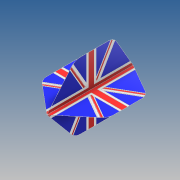
# Autodesk Inventor part: Millan Dart Flight
Saved by Autodesk Inventor 2018.2 (Build 222227000, 227)
## iProperties
Created: 2018-01-12
Part Number: Millan Dart Flight
Material: Generic
Document SubType Name: Modeling
Designer: Thomas Savage
Density: 1 g/cm^3
Appearance: Default
Author: Thomas Savage
Autodesk Inventor part; units mm, degrees
ref_plane "YZ Plane" through (0, 0, 0) normal (1, 0, 0) x (0, 1, 0)
ref_plane "XZ Plane" through (0, 0, 0) normal (0, 1, 0) x (-1, 0, 0)
ref_plane "XY Plane" through (0, 0, 0) normal (0, 0, 1) x (1, 0, 0)
sketch "Sketch1" plane through (0, 0, 0) normal (0, 0, 1) x (1, 0, 0)
  line L0 (0, 22) -> (0, -22)
  line L1 (0, 22) -> (17, 12.185)
  line L2 (17, 12.185) -> (17, -7.7353)
  line L3 (17, -7.7353) -> (0, -22)
  point P0 (0, 0)
  point P1 (0, 0)
  dimension "d0" = 44
  dimension "d1" = 17
  dimension "d3" = 60
  dimension "d4" = 50
  constraints: 8 end point, 2 vertical, 1 coincident, 1 midpoint, 1 vertical alignment
  measures "d0" distance of L0.start L0.end
  measures "d1" distance between parallel lines of L0 L2
  measures "d3" angle of L1 L0
  measures "d4" angle of L0 L3
extrude "Extrusion1" add sketch "Sketch1" along normal blind 0.01
fillet "Fillet1" radius 5 1 edges at (17, 12.185, 0.005)
fillet "Fillet2" radius 6 1 edges at (17, -7.7353, 0.005)
pattern_circular "Circular Pattern1" count 4 over 360 about axis through (0, -10, 0) along (0, 1, 0) of "Extrusion1", "Fillet1", "Fillet2"
sketch "Sketch2" plane through (0, 0, 0) normal (0, 0, -1) x (-1, 0, 0)
  line L0 (-0.01, -21.9916) -> (-0.01, 21.9942) projected
  line L1 (-14.5, 13.6284) -> (-0.01, 21.9942) projected
  arc A0 (-14.5, 13.6284) -> (-17, 9.2983) centre (-12, 9.2983) ccw projected
  line L2 (-17, -4.9375) -> (-17, 9.2983) projected
  arc A1 (-17, -4.9375) -> (-14.8567, -9.5337) centre (-11, -4.9375) ccw projected
  line L3 (-0.01, -21.9916) -> (-14.8567, -9.5337) projected
  line L4 (-0.01, 13.6284) -> (-0.01, 22) projected
  line L5 (-1.51, 21.1282) -> (-1.51, 2.1804)
  line L6 (-1.51, 2.1804) -> (-17, 2.1804)
  line L7 (-17, -0.8196) -> (-1.51, -0.8196)
  line L8 (-1.51, -0.8196) -> (-1.51, -20.733)
  line L9 (-2.51, 20.5509) -> (-2.51, 3.1804)
  line L10 (-2.51, 3.1804) -> (-17, 3.1804)
  line L11 (-17, -1.8196) -> (-2.51, -1.8196)
  line L12 (-2.51, -1.8196) -> (-2.51, -19.8939)
  line L13 (-2.51, 5.201) -> (-15.606, 12.7619)
  line L14 (-4.01, 3.1804) -> (-16.8321, 10.5832)
  line L15 (-4.01, -1.8196) -> (-15.7529, -8.5994)
  line L16 (-2.51, -3.7171) -> (-13.9306, -10.3108)
  line L17 (-3.41, 3.1804) -> (-16.7437, 10.8786)
  line L18 (-2.51, 3.8155) -> (-16.3317, 11.7955)
  line L19 (-2.51, -3.3707) -> (-14.1752, -10.1056)
  line L20 (-2.51, -2.216) -> (-14.9881, -9.4202)
  line L21 (-17, -4.9375) -> (-17, 9.2983) projected
  point P0 (0, 0)
  dimension "d13" = 1.5
  dimension "d15" = 3
  dimension "d16" = 4.1179
  dimension "d17" = 1
  dimension "d18" = 1
  dimension "d20" = 30
  dimension "d21" = 1
  dimension "d22" = 30
  dimension "d23" = 1
  dimension "d24" = 2.5
  dimension "d25" = 2.5
  dimension "d26" = 1.5
  dimension "d27" = 1.5
  dimension "d28" = 0.3
  dimension "d29" = 1
  dimension "d30" = 0.3
  dimension "d31" = 1
  constraints: 32 end point, 19 point on line, 7 parallel, 6 point on circle, 1 midpoint, 1 vertical
  measures "d13" distance between parallel lines of L0 L5
  measures "d15" distance between parallel lines of L7 L6
  measures "d16" distance of L2.start L7.start
  measures "d17" distance between parallel lines of L5 L9
  measures "d18" distance between parallel lines of L7 L11
  measures "d20" angle of L10 L14
  measures "d21" distance between parallel lines of L6 L10
  measures "d22" angle of L11 L15
  measures "d23" distance between parallel lines of L8 L12
  measures "d24" distance of L13.end L14.end
  measures "d25" distance of L15.end L16.end
  measures "d26" distance of L11.end L15.start
  measures "d27" distance of L9.end L14.start
  measures "d28" distance between parallel lines of L14 L17
  measures "d29" distance between parallel lines of L17 L18
  measures "d30" distance between parallel lines of L16 L19
  measures "d31" distance between parallel lines of L19 L20
sketch "Sketch3" plane through (0.01, -21.9916, 0) normal (1, 0, 0) x (0, 0, -1)
  arc A0 (14.8567, 12.4579) -> (17, 17.0541) centre (11, 17.0541) ccw projected
  line L0 (17, 17.0541) -> (17, 31.2899) projected
  arc A1 (17, 31.2899) -> (14.5, 35.62) centre (12, 31.2899) ccw projected
  line L1 (14.5, 35.62) -> (0, 43.9916) projected
  line L2 (0, 43.9916) -> (0, 43.9858) projected
  line L3 (0, 0) -> (0, 43.9858) projected
  line L4 (0, 0) -> (0, -0.0084) projected
  line L5 (0, -0.0084) -> (14.8567, 12.4579) projected
  line L6 (1.5, 43.1256) -> (1.5, 24.1721)
  line L7 (1.5, 24.1721) -> (17, 24.1721)
  line L8 (1.5, 1.2503) -> (1.5, 21.1721)
  line L9 (1.5, 21.1721) -> (17, 21.1721)
  line L10 (2.5, 42.5482) -> (2.5, 25.1721)
  line L11 (2.5, 25.1721) -> (17, 25.1721)
  line L12 (17, 20.1721) -> (2.5, 20.1721)
  line L13 (2.5, 20.1721) -> (2.5, 2.0894)
  line L14 (2.5, 27.1927) -> (15.6023, 34.7574)
  line L15 (4, 25.1721) -> (16.8307, 32.58)
  line L16 (4, 20.1721) -> (15.7499, 13.3883)
  line L17 (2.5, 18.2749) -> (13.9269, 11.6776)
  line L18 (2.5, 26.8463) -> (15.8083, 34.5298)
  line L19 (2.5, 25.6916) -> (16.3784, 33.7043)
  line L20 (3.4, 20.1721) -> (15.5583, 13.1526)
  line L21 (2.5, 19.5371) -> (14.8179, 12.4253)
  point P0 (0, 21.9916)
  dimension "d32" = 1.5
  dimension "d33" = 3
  dimension "d34" = 4.118
  dimension "d35" = 1
  dimension "d36" = 1
  dimension "d37" = 1
  dimension "d38" = 1
  dimension "d39" = 30
  dimension "d40" = 30
  dimension "d41" = 2.5
  dimension "d42" = 1.5
  dimension "d43" = 2.5
  dimension "d44" = 1.5
  dimension "d45" = 0.3
  dimension "d46" = 1
  dimension "d47" = 0.3
  dimension "d48" = 1
  constraints: 32 end point, 20 point on line, 6 parallel, 6 point on circle, 2 perpendicular, 1 vertical
  measures "d32" distance between parallel lines of L3 L6
  measures "d33" distance between parallel lines of L9 L7
  measures "d34" distance of L0.start L9.end
  measures "d35" distance between parallel lines of L6 L10
  measures "d36" distance between parallel lines of L9 L12
  measures "d37" distance between parallel lines of L7 L11
  measures "d38" distance between parallel lines of L13 L8
  measures "d39" angle of L11 L15
  measures "d40" angle of L12 L16
  measures "d41" distance of L15.end L14.end
  measures "d42" distance of L10.end L15.start
  measures "d43" distance of L16.end L17.end
  measures "d44" distance of L12.end L16.start
  measures "d45" distance between parallel lines of L14 L18
  measures "d46" distance between parallel lines of L18 L19
  measures "d47" distance between parallel lines of L16 L20
  measures "d48" distance between parallel lines of L20 L21
extrude "Extrusion2" add sketch "Sketch2" along normal blind 0.01 separate body contours L3 L8 L7 L2 L6 L5 L1 L0 | L3 A1 L20 L12 L19 | L9 L10 L17 A0 L18
extrude "Extrusion3" add sketch "Sketch2" along normal blind 0.01 separate body contours L3 L12 L11 L2 L7 L8 | L5 L6 L2 L10 L9 L1 | L3 L19 L12 L16 | L9 L18 A0 L13 | L20 A1 L15 L11 L12 | L14 A0 L17 L10
extrude "Extrusion4" add sketch "Sketch3" along normal blind 0.01 separate body contours L5 L21 L13 L12 L20 A0 | L5 L4 L3 L2 L1 L6 L7 L0 L9 L8 | L19 L10 L18 A1
extrude "Extrusion5" add sketch "Sketch3" along normal blind 0.01 separate body contours L20 L12 L16 A0 | L5 L17 L13 L21 | L12 L13 L5 L8 L9 L0 | L7 L6 L1 L10 L11 L0 | L11 L10 L19 A1 L15 | L14 A1 L18 L10
pattern_circular "Circular Pattern5" count 4 over 360 about axis through (0, -10, 0) along (0, 1, 0) of "Extrusion2" bodies 2
pattern_circular "Circular Pattern6" count 4 over 360 about axis through (0, -10, 0) along (0, 1, 0) of "Extrusion3" bodies 3
pattern_circular "Circular Pattern7" count 4 over 360 about axis through (0, -10, 0) along (0, 1, 0) of "Extrusion4" bodies 4
pattern_circular "Circular Pattern8" count 4 over 360 about axis through (0, -10, 0) along (0, 1, 0) of "Extrusion5" bodies 5
sketch "Sketch4" plane through (0, 0, 0) normal (0, 0, -1) x (-1, 0, 0)
  line L0 (16.3784, 11.7127) -> (2.5, 3.7) projected
  line L1 (-2.51, 5.201) -> (-15.606, 12.7619) projected
  line L2 (-2.51, 20.5509) -> (-2.51, 5.201) projected
  arc A0 (-14.5, 13.6284) -> (-17, 9.2983) centre (-12, 9.2983) ccw projected
  line L3 (-14.5, 13.6284) -> (-0.01, 21.9942) projected
  line L4 (-4.01, 3.1804) -> (-17, 3.1804) projected
  line L5 (-16.8321, 10.5832) -> (-4.01, 3.1804) projected
  line L6 (-17, -4.9375) -> (-17, 9.2983) projected
  line L7 (-17, -1.8196) -> (-4.01, -1.8196) projected
  line L8 (-4.01, -1.8196) -> (-15.7529, -8.5994) projected
  arc A1 (-17, -4.9375) -> (-14.8567, -9.5337) centre (-11, -4.9375) ccw projected
  line L9 (-13.9306, -10.3108) -> (-2.51, -3.7171) projected
  line L10 (-2.51, -3.7171) -> (-2.51, -19.8939) projected
  line L11 (-0.01, -21.9916) -> (-14.8567, -9.5337) projected
  point P0 (0, 0)
extrude "Extrusion6" add sketch "Sketch4" along normal blind 0.01 separate body
sketch "Sketch5" plane through (0.01, -21.9916, 0) normal (1, 0, 0) x (0, 0, -1)
  line L0 (14.5, 35.62) -> (0, 43.9916) projected
  arc A0 (17, 31.2899) -> (14.5, 35.62) centre (12, 31.2899) ccw projected
  line L1 (2.5, 27.1927) -> (2.5, 42.5482) projected
  line L2 (15.6023, 34.7574) -> (2.5, 27.1927) projected
  line L3 (4, 25.1721) -> (16.8307, 32.58) projected
  line L4 (17, 25.1721) -> (4, 25.1721) projected
  line L5 (17, 17.0541) -> (17, 31.2899) projected
  line L6 (4, 20.1721) -> (17, 20.1721) projected
  line L7 (15.7499, 13.3883) -> (4, 20.1721) projected
  arc A1 (14.8567, 12.4579) -> (17, 17.0541) centre (11, 17.0541) ccw projected
  line L8 (2.5, 18.2749) -> (13.9269, 11.6776) projected
  line L9 (0, -0.0084) -> (14.8567, 12.4579) projected
  line L10 (2.5, 2.0894) -> (2.5, 18.2749) projected
  point P0 (0, 21.9916)
extrude "Extrusion7" add sketch "Sketch5" along normal blind 0.01 separate body
pattern_circular "Circular Pattern9" count 4 over 360 about axis through (0, -10, 0) along (0, 1, 0) of "Extrusion6" bodies 6
pattern_circular "Circular Pattern10" count 4 over 360 about axis through (0, -10, 0) along (0, 1, 0) of "Extrusion7" bodies 7
body "Solid1"
body "Solid2"
body "Solid3"
body "Solid4"
body "Solid5"
body "Solid6"
body "Solid7"
